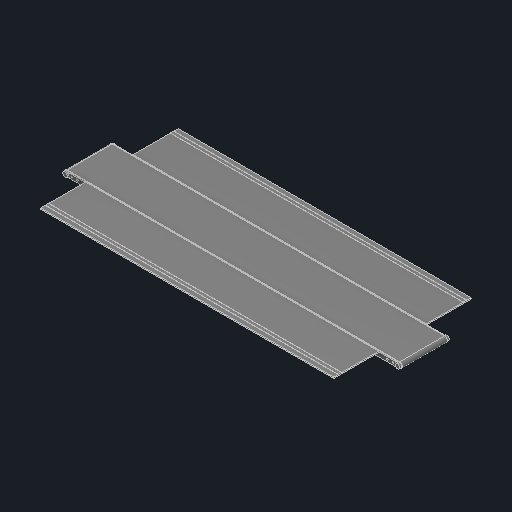
# Autodesk Inventor part: SACMI DPA CARDBOARD CONVEYOR
Saved by Autodesk Inventor 2025 (Build 290162000, 162)
## iProperties
Created: 2024-05-26
Part Number: SACMI DPA CARDBOARD CONVEYOR
Material: Generic
Document SubType Name: Modeling
Designer: zulet
Density: 1 g/cm^3
Appearance: Smooth - Black
Author: zulet
Autodesk Inventor part; units mm, degrees
ref_plane "YZ Plane" through (0, 0, 0) normal (1, 0, 0) x (0, 1, 0)
ref_plane "XZ Plane" through (0, 0, 0) normal (0, 1, 0) x (-1, 0, 0)
ref_plane "XY Plane" through (0, 0, 0) normal (0, 0, 1) x (1, 0, 0)
sketch "Sketch1" plane through (0, 0, 0) normal (0, 0, 1) x (1, 0, 0)
  line L0 (-1500, 0) -> (1500, 0) construction
  line L1 (-1475, -25) -> (1475, -25)
  line L2 (1475, 25) -> (-1475, 25)
  arc A0 (-1475, 25) -> (-1475, -25) centre (-1475, 0) ccw
  arc A1 (1475, -25) -> (1475, 25) centre (1475, 0) ccw
  line L3 (-1475, 20) -> (1475, 20)
  arc A2 (1475, -20) -> (1475, 20) centre (1475, 0) ccw
  line L4 (1475, -20) -> (-1475, -20)
  arc A3 (-1475, 20) -> (-1475, -20) centre (-1475, 0) ccw
  circle A4 centre (-1475, 0) radius 20
  circle A5 centre (1475, 0) radius 20
  circle A6 centre (-1425, 0) radius 4.4168
  circle A7 centre (-1375, 0) radius 5.9739
  circle A8 centre (-1449.8431, 13.9793) radius 1.9266
  circle A9 centre (-1449.8431, -14.2029) radius 1.6337
  circle A10 centre (1450.3444, 13.9793) radius 2.1646
  circle A11 centre (1450.3444, -14.2029) radius 2.7119
  circle A12 centre (1425, 0) radius 6.6221
  circle A13 centre (1375, 0) radius 8.5174
  point P0 (0, 0)
  point P1 (0, 0)
  point P2 (1500, 0)
  point P3 (-1500, 0)
  dimension "d0" = 3000
  dimension "d1" = 50
  dimension "d2" = 5
  dimension "d17" = 75
  dimension "d18" = 50
  dimension "d19" = 75
  dimension "d20" = 50
  constraints: 12 centre point, 12 end point, 12 point on circle, 6 point on line, 4 tangent, 3 coincident, 2 parallel, 1 horizontal, 1 midpoint, 9 other
  measures "d0" distance of L0.start L0.end
  measures "d1" diameter of A1
  measures "d2" distance between parallel lines of L2 L3
  measures "d17" distance of point (1500, 0) A12.centre
  measures "d18" distance of A12.centre A13.centre
  measures "d19" distance of point (-1500, 0) A6.centre
  measures "d20" distance of A7.centre A6.centre
extrude "Extrusion1" add sketch "Sketch1" along normal mid plane 400 contours A0 L2 A1 L1
extrude "Extrusion2" add sketch "Sketch1" along normal mid plane 420 contours L3 A5 L4 A4
extrude "Extrusion3" add sketch "Sketch1" along normal mid plane 440 contours A4 A3 | A2 A5
sketch "Sketch2" plane through (-1475, 25, 200) normal (0, 1, 0) x (1, 0, 0)
  line L0 (0, 410) -> (2950, 410) projected
  line L1 (175, 410) -> (2775, 410)
  line L2 (2775, 410) -> (2775, 810)
  line L3 (2775, 810) -> (175, 810)
  line L4 (175, 810) -> (175, 410)
  line L5 (175, 770) -> (2775, 770)
  line L6 (2775, 770) -> (2775, 740)
  line L7 (2775, 740) -> (175, 740)
  line L8 (175, 740) -> (175, 770)
  line L9 (2950, 400) -> (2950, 0) construction
  line L10 (2950, 200) -> (0, 200) construction
  line L11 (0, 400) -> (0, 0) construction
  line L12 (175, -10) -> (2775, -10)
  line L13 (2775, -10) -> (2775, -410)
  line L14 (2775, -410) -> (175, -410)
  line L15 (175, -410) -> (175, -10)
  line L16 (175, -370) -> (2775, -370)
  line L17 (2775, -370) -> (2775, -340)
  line L18 (2775, -340) -> (175, -340)
  line L19 (175, -340) -> (175, -370)
  point P0 (1475, 200)
  point P1 (1475, 410)
  point P2 (1475, -10)
  point P3 (175, -340)
  point P4 (175, 740)
  dimension "d9" = 2600
  dimension "d10" = 400
  dimension "d11" = 30
  dimension "d12" = 40
  constraints: 34 end point, 9 symmetric about line, 5 point on line, 4 midpoint, 4 parallel, 2 horizontal, 2 perpendicular
  measures "d9" distance of L3.end L2.end
  measures "d10" distance of L2.end L1.end
  measures "d11" distance between parallel lines of L5 L7
  measures "d12" distance between parallel lines of L3 L5
extrude "Extrusion4" add sketch "Sketch2" against normal blind 10
extrude "Extrusion5" add sketch "Sketch2" along normal blind 2 contours L4 L5 L2 L7 | L18 L13 L16 L15
body "Solid1"
